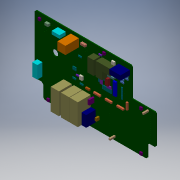
# Autodesk Inventor part: E99245-1178
Saved by Autodesk Inventor 2018 (Build 220105000, 105)
## iProperties
Created: 2004-11-23
Part Number: E99245-1178
Document SubType Name: Modeling
Designer: Autodesk, Inc.
Manufacturer: Standard
Standards Organization: Custom
Description: CONTROLER CARD, 29 SERIES
Engineer: N. GINEER
Mass: 79.5696 g
Surface Area: 565.686 cm^2
Volume: 79.5696 cm^3
Density: 1 g/cm^3
Material: Generic
Appearance: Board Outline
CAGE: 1LJX3
Dept. ID: Product Design
Description #2: ---
Finish #1: ---
Finish #2: ---
Material ID: ---
Project Number: ---
Author: Autodesk, Inc.
Autodesk Inventor part; units mm, degrees
ref_plane "YZ Plane" through (0, 0, 0) normal (1, 0, 0) x (0, 1, 0)
ref_plane "XZ Plane" through (0, 0, 0) normal (0, 1, 0) x (-1, 0, 0)
ref_plane "XY Plane" through (0, 0, 0) normal (0, 0, 1) x (1, 0, 0)
sketch "Sketch1" plane through (0, 0, 0) normal (0, 0, 1) x (1, 0, 0)
  line L0 (181.9999, 1.9998) -> (181.9999, 20)
  line L1 (181.9999, 20) -> (185.0001, 23.0001)
  line L2 (185.0001, 23.0001) -> (194.0001, 23.0001)
  line L3 (194.0001, 23.0001) -> (195.9999, 25)
  line L4 (195.9999, 25) -> (195.9999, 69.9999)
  line L5 (195.9999, 69.9999) -> (194.0001, 72.0001)
  line L6 (194.0001, 72.0001) -> (158.4998, 72.0001)
  arc A0 (156.9999, 73.5) -> (158.4998, 72.0001) centre (158.4998, 73.5) ccw
  line L7 (156.9999, 73.5) -> (156.9999, 116.0001)
  line L8 (156.9999, 116.0001) -> (155.0001, 117.9999)
  line L9 (155.0001, 117.9999) -> (1.9998, 117.9999)
  line L10 (1.9998, 117.9999) -> (0, 116.0001)
  line L11 (0, 116.0001) -> (0, 25)
  line L12 (0, 25) -> (1.9998, 23.0001)
  line L13 (1.9998, 23.0001) -> (10.9999, 23.0001)
  line L14 (10.9999, 23.0001) -> (14.0001, 20)
  line L15 (14.0001, 20) -> (14.0001, 1.9998)
  line L16 (14.0001, 1.9998) -> (15.9999, 0)
  line L17 (15.9999, 0) -> (180.0001, 0)
  line L18 (180.0001, 0) -> (181.9999, 1.9998)
  circle A1 centre (22.987, 3.9878) radius 1.7526
  circle A2 centre (172.9994, 3.9878) radius 1.7526
  circle A3 centre (172.9994, 66.9798) radius 1.7526
  circle A4 centre (113.0046, 113.9952) radius 1.7526
  circle A5 centre (8.9916, 110.0074) radius 1.7526
  circle A6 centre (137.3124, 106.68) radius 0.508
  circle A7 centre (152.2476, 106.68) radius 0.508
  circle A8 centre (103.505, 19.685) radius 0.3937
  circle A9 centre (103.505, 17.145) radius 0.3937
  circle A10 centre (94.615, 25.8826) radius 0.508
  circle A11 centre (94.615, 10.9474) radius 0.508
  circle A12 centre (83.82, 41.275) radius 0.4826
  circle A13 centre (83.82, 12.065) radius 0.4826
  circle A14 centre (95.25, 42.545) radius 0.3937
  circle A15 centre (95.25, 37.465) radius 0.3937
  circle A16 centre (69.85, 41.275) radius 0.4826
  circle A17 centre (69.85, 12.065) radius 0.4826
  circle A18 centre (61.595, 17.145) radius 0.3937
  circle A19 centre (61.595, 12.065) radius 0.3937
  circle A20 centre (53.34, 41.275) radius 0.4826
  circle A21 centre (53.34, 12.065) radius 0.4826
  circle A22 centre (100.33, 109.22) radius 0.635
  circle A23 centre (100.33, 78.74) radius 0.635
  circle A24 centre (106.045, 100.965) radius 0.635
  circle A25 centre (136.525, 100.965) radius 0.635
  circle A26 centre (113.665, 109.855) radius 0.635
  circle A27 centre (113.665, 79.375) radius 0.635
  circle A28 centre (62.23, 107.315) radius 0.4318
  circle A29 centre (67.31, 107.315) radius 0.4318
  circle A30 centre (120.65, 107.95) radius 0.3556
  circle A31 centre (120.65, 97.79) radius 0.3556
  circle A32 centre (73.66, 110.49) radius 0.5334
  circle A33 centre (87.63, 110.49) radius 0.5334
  circle A34 centre (16.51, 109.855) radius 0.508
  circle A35 centre (27.94, 109.855) radius 0.508
  circle A36 centre (55.245, 109.855) radius 0.7112
  circle A37 centre (50.165, 109.855) radius 0.7112
  circle A38 centre (37.465, 109.855) radius 0.7112
  circle A39 centre (32.385, 109.855) radius 0.7112
  circle A40 centre (127, 81.28) radius 0.4318
  circle A41 centre (127, 78.74) radius 0.4318
  circle A42 centre (127, 76.2) radius 0.4318
  circle A43 centre (127, 73.66) radius 0.4318
  circle A44 centre (127, 71.12) radius 0.4318
  circle A45 centre (127, 68.58) radius 0.4318
  circle A46 centre (127, 66.04) radius 0.4318
  circle A47 centre (134.62, 66.04) radius 0.4318
  circle A48 centre (134.62, 68.58) radius 0.4318
  circle A49 centre (134.62, 71.12) radius 0.4318
  circle A50 centre (134.62, 73.66) radius 0.4318
  circle A51 centre (134.62, 76.2) radius 0.4318
  circle A52 centre (134.62, 78.74) radius 0.4318
  circle A53 centre (134.62, 81.28) radius 0.4318
  circle A54 centre (115.57, 81.915) radius 0.4318
  circle A55 centre (115.57, 79.375) radius 0.4318
  circle A56 centre (115.57, 76.835) radius 0.4318
  circle A57 centre (115.57, 74.295) radius 0.4318
  circle A58 centre (123.19, 74.295) radius 0.4318
  circle A59 centre (123.19, 76.835) radius 0.4318
  circle A60 centre (123.19, 79.375) radius 0.4318
  circle A61 centre (123.19, 81.915) radius 0.4318
  circle A62 centre (129.413, 5.715) radius 0.4699
  circle A63 centre (183.515, 68.58) radius 0.4699
  circle A64 centre (126.365, 92.71) radius 0.4699
  circle A65 centre (131.445, 92.71) radius 0.4699
  circle A66 centre (133.985, 92.71) radius 0.4699
  circle A67 centre (186.69, 62.865) radius 0.4699
  circle A68 centre (186.69, 60.325) radius 0.4699
  circle A69 centre (186.69, 57.785) radius 0.4699
  circle A70 centre (186.69, 55.245) radius 0.4699
  circle A71 centre (186.69, 52.705) radius 0.4699
  circle A72 centre (186.69, 50.165) radius 0.4699
  circle A73 centre (186.69, 47.625) radius 0.4699
  circle A74 centre (186.69, 45.085) radius 0.4699
  circle A75 centre (186.69, 42.545) radius 0.4699
  circle A76 centre (186.69, 40.005) radius 0.4699
  circle A77 centre (186.69, 37.465) radius 0.4699
  circle A78 centre (186.69, 34.925) radius 0.4699
  circle A79 centre (186.69, 32.385) radius 0.4699
  circle A80 centre (186.69, 29.845) radius 0.4699
  circle A81 centre (81.915, 51.435) radius 0.3937
  circle A82 centre (92.075, 51.435) radius 0.3937
  circle A83 centre (147.32, 51.435) radius 0.4318
  circle A84 centre (132.08, 51.435) radius 0.4318
  circle A85 centre (128.27, 51.435) radius 0.4318
  circle A86 centre (113.03, 51.435) radius 0.4318
  circle A87 centre (109.855, 51.435) radius 0.4318
  circle A88 centre (94.615, 51.435) radius 0.4318
  circle A89 centre (150.495, 51.435) radius 0.4318
  circle A90 centre (150.495, 66.675) radius 0.4318
  circle A91 centre (120.65, 5.715) radius 0.3937
  circle A92 centre (120.65, 15.875) radius 0.3937
  circle A93 centre (138.43, 66.04) radius 0.4318
  circle A94 centre (138.43, 81.28) radius 0.4318
  circle A95 centre (101.6, 66.04) radius 0.4318
  circle A96 centre (101.6, 81.28) radius 0.4318
  circle A97 centre (120.65, 19.685) radius 0.3937
  circle A98 centre (120.65, 29.845) radius 0.3937
  circle A99 centre (60.325, 66.04) radius 0.3937
  circle A100 centre (60.325, 76.2) radius 0.3937
  circle A101 centre (120.65, 33.02) radius 0.3937
  circle A102 centre (120.65, 43.18) radius 0.3937
  circle A103 centre (117.475, 43.18) radius 0.3937
  circle A104 centre (107.315, 43.18) radius 0.3937
  circle A105 centre (8.255, 27.94) radius 0.4318
  circle A106 centre (8.255, 53.34) radius 0.4318
  circle A107 centre (26.7462, 23.495) radius 0.6604
  circle A108 centre (39.243, 23.495) radius 0.6604
  circle A109 centre (39.243, 28.4734) radius 0.6604
  circle A110 centre (26.7462, 28.4734) radius 0.6604
  circle A111 centre (32.9946, 30.48) radius 0.9144
  circle A112 centre (32.9946, 21.4884) radius 0.9144
  circle A113 centre (106.68, 85.09) radius 0.6604
  circle A114 centre (137.16, 85.09) radius 0.6604
  circle A115 centre (144.78, 73.66) radius 0.6604
  circle A116 centre (137.16, 62.23) radius 0.6604
  circle A117 centre (106.68, 62.23) radius 0.6604
  circle A118 centre (99.06, 73.66) radius 0.6604
  circle A119 centre (32.9946, 73.9902) radius 4.7498
  circle A120 centre (113.665, 102.235) radius 0.3048
  circle A121 centre (167.7416, 62.8904) radius 0.3048
  circle A122 centre (151.13, 86.36) radius 0.3048
  circle A123 centre (78.105, 66.04) radius 0.3048
  circle A124 centre (92.075, 96.52) radius 0.3048
  circle A125 centre (71.755, 53.34) radius 0.3048
  circle A126 centre (69.215, 72.39) radius 0.3048
  circle A127 centre (69.215, 74.93) radius 0.3048
  circle A128 centre (139.065, 64.135) radius 0.3048
  circle A129 centre (69.85, 67.31) radius 0.3048
  circle A130 centre (115.57, 71.755) radius 0.3048
  circle A131 centre (60.96, 62.865) radius 0.3048
  circle A132 centre (71.755, 67.31) radius 0.3048
  circle A133 centre (60.96, 60.325) radius 0.3048
  circle A134 centre (71.12, 55.88) radius 0.3048
  circle A135 centre (72.39, 71.755) radius 0.3048
  circle A136 centre (14.605, 27.94) radius 0.3048
  circle A137 centre (48.26, 101.6) radius 0.3048
  circle A138 centre (36.195, 91.44) radius 0.3048
  circle A139 centre (111.125, 108.585) radius 0.3048
  circle A140 centre (55.5752, 102.5144) radius 0.3048
  circle A141 centre (77.47, 97.79) radius 0.3048
  circle A142 centre (15.875, 95.885) radius 0.6858
  circle A143 centre (15.875, 100.965) radius 0.6858
  circle A144 centre (18.415, 98.425) radius 0.6858
  circle A145 centre (81.915, 100.33) radius 0.6858
  circle A146 centre (81.915, 105.41) radius 0.6858
  circle A147 centre (84.455, 102.87) radius 0.6858
  constraints: 148 centre point, 38 end point, 2 point on circle
extrude "example2.max_Outline" add sketch "Sketch1" along normal blind 1.5748
sketch "3.5MTH, 0_1" plane through (0, 0, 1.5748) normal (0, 0, 1) x (1, 0, 0)
  line L0 (21.082, 2.0828) -> (21.082, 5.8928)
  line L1 (21.082, 5.8928) -> (24.892, 5.8928)
  line L2 (24.892, 5.8928) -> (24.892, 2.0828)
  line L3 (24.892, 2.0828) -> (21.082, 2.0828)
  constraints: 8 end point
extrude "11_2" add sketch "3.5MTH, 0_1" along normal blind 2.54
sketch "3.5MTH, 0_3" plane through (0, 0, 1.5748) normal (0, 0, 1) x (1, 0, 0)
  line L0 (171.0944, 2.0828) -> (171.0944, 5.8928)
  line L1 (171.0944, 5.8928) -> (174.9044, 5.8928)
  line L2 (174.9044, 5.8928) -> (174.9044, 2.0828)
  line L3 (174.9044, 2.0828) -> (171.0944, 2.0828)
  constraints: 8 end point
extrude "21_4" add sketch "3.5MTH, 0_3" along normal blind 2.54
sketch "3.5MTH, 0_5" plane through (0, 0, 1.5748) normal (0, 0, 1) x (1, 0, 0)
  line L0 (171.0944, 65.0748) -> (171.0944, 68.8848)
  line L1 (171.0944, 68.8848) -> (174.9044, 68.8848)
  line L2 (174.9044, 68.8848) -> (174.9044, 65.0748)
  line L3 (174.9044, 65.0748) -> (171.0944, 65.0748)
  constraints: 8 end point
extrude "31_6" add sketch "3.5MTH, 0_5" along normal blind 2.54
sketch "3.5MTH, 0_7" plane through (0, 0, 1.5748) normal (0, 0, 1) x (1, 0, 0)
  line L0 (111.0996, 112.0902) -> (111.0996, 115.9002)
  line L1 (111.0996, 115.9002) -> (114.9096, 115.9002)
  line L2 (114.9096, 115.9002) -> (114.9096, 112.0902)
  line L3 (114.9096, 112.0902) -> (111.0996, 112.0902)
  constraints: 8 end point
extrude "41_8" add sketch "3.5MTH, 0_7" along normal blind 2.54
sketch "3.5MTH, 0_9" plane through (0, 0, 1.5748) normal (0, 0, 1) x (1, 0, 0)
  line L0 (7.0866, 108.1024) -> (7.0866, 111.9124)
  line L1 (7.0866, 111.9124) -> (10.8966, 111.9124)
  line L2 (10.8966, 111.9124) -> (10.8966, 108.1024)
  line L3 (10.8966, 108.1024) -> (7.0866, 108.1024)
  constraints: 8 end point
extrude "51_10" add sketch "3.5MTH, 0_9" along normal blind 2.54
sketch "RAD_.725X.300_LS.588_.040, 470NF_11" plane through (0, 0, 1.5748) normal (0, 0, 1) x (1, 0, 0)
  line L0 (153.67, 110.49) -> (135.89, 110.49)
  line L1 (135.89, 110.49) -> (135.89, 102.87)
  line L2 (135.89, 102.87) -> (153.67, 102.87)
  line L3 (153.67, 102.87) -> (153.67, 110.49)
  constraints: 8 end point
extrude "C1_12" add sketch "RAD_.725X.300_LS.588_.040, 470NF_11" along normal blind 15.24
sketch "SM_C_1206, 10NF_13" plane through (0, 0, 1.5748) normal (0, 0, 1) x (1, 0, 0)
  line L0 (117.602, 62.865) -> (119.888, 62.865)
  line L1 (119.888, 62.865) -> (119.888, 68.453)
  line L2 (119.888, 68.453) -> (117.602, 68.453)
  line L3 (117.602, 68.453) -> (117.602, 62.865)
  constraints: 8 end point
extrude "C2_14" add sketch "SM_C_1206, 10NF_13" along normal blind 1.27
sketch "SM_C_1206, 10NF_15" plane through (0, 0, 1.5748) normal (0, 0, 1) x (1, 0, 0)
  line L0 (105.918, 75.565) -> (103.632, 75.565)
  line L1 (103.632, 75.565) -> (103.632, 69.977)
  line L2 (103.632, 69.977) -> (105.918, 69.977)
  line L3 (105.918, 69.977) -> (105.918, 75.565)
  constraints: 8 end point
extrude "C3_16" add sketch "SM_C_1206, 10NF_15" along normal blind 1.27
sketch "SM_C_1206, 10NF_17" plane through (0, 0, 1.5748) normal (0, 0, 1) x (1, 0, 0)
  line L0 (112.268, 68.58) -> (109.982, 68.58)
  line L1 (109.982, 68.58) -> (109.982, 62.992)
  line L2 (109.982, 62.992) -> (112.268, 62.992)
  line L3 (112.268, 62.992) -> (112.268, 68.58)
  constraints: 8 end point
extrude "C4_18" add sketch "SM_C_1206, 10NF_17" along normal blind 1.27
sketch "SM_C_1206, 10NF_19" plane through (0, 0, 1.5748) normal (0, 0, 1) x (1, 0, 0)
  line L0 (115.062, 62.865) -> (117.348, 62.865)
  line L1 (117.348, 62.865) -> (117.348, 68.453)
  line L2 (117.348, 68.453) -> (115.062, 68.453)
  line L3 (115.062, 68.453) -> (115.062, 62.865)
  constraints: 8 end point
extrude "C5_20" add sketch "SM_C_1206, 10NF_19" along normal blind 1.27
sketch "SM_C_1206, 10NF_21" plane through (0, 0, 1.5748) normal (0, 0, 1) x (1, 0, 0)
  line L0 (62.23, 70.993) -> (62.23, 68.707)
  line L1 (62.23, 68.707) -> (67.818, 68.707)
  line L2 (67.818, 68.707) -> (67.818, 70.993)
  line L3 (67.818, 70.993) -> (62.23, 70.993)
  constraints: 8 end point
extrude "C6_22" add sketch "SM_C_1206, 10NF_21" along normal blind 1.27
sketch "SM_C_1206, 10NF_23" plane through (0, 0, 1.5748) normal (0, 0, 1) x (1, 0, 0)
  line L0 (62.23, 68.453) -> (62.23, 66.167)
  line L1 (62.23, 66.167) -> (67.818, 66.167)
  line L2 (67.818, 66.167) -> (67.818, 68.453)
  line L3 (67.818, 68.453) -> (62.23, 68.453)
  constraints: 8 end point
extrude "C7_24" add sketch "SM_C_1206, 10NF_23" along normal blind 1.27
sketch "SM_C_1206, 10NF_25" plane through (0, 0, 1.5748) normal (0, 0, 1) x (1, 0, 0)
  line L0 (73.66, 53.213) -> (73.66, 50.927)
  line L1 (73.66, 50.927) -> (79.248, 50.927)
  line L2 (79.248, 50.927) -> (79.248, 53.213)
  line L3 (79.248, 53.213) -> (73.66, 53.213)
  constraints: 8 end point
extrude "C8_26" add sketch "SM_C_1206, 10NF_25" along normal blind 1.27
sketch "SM_C_1206, 10NF_27" plane through (0, 0, 1.5748) normal (0, 0, 1) x (1, 0, 0)
  line L0 (136.017, 95.885) -> (138.303, 95.885)
  line L1 (138.303, 95.885) -> (138.303, 101.473)
  line L2 (138.303, 101.473) -> (136.017, 101.473)
  line L3 (136.017, 101.473) -> (136.017, 95.885)
  constraints: 8 end point
extrude "C9_28" add sketch "SM_C_1206, 10NF_27" along normal blind 1.27
sketch "RAD_.150X.100_LS.100_.031, 1NF_29" plane through (0, 0, 1.5748) normal (0, 0, 1) x (1, 0, 0)
  line L0 (102.1334, 20.7264) -> (102.1334, 16.1036)
  line L1 (102.1334, 16.1036) -> (104.8766, 16.1036)
  line L2 (104.8766, 16.1036) -> (104.8766, 20.7264)
  line L3 (104.8766, 20.7264) -> (102.1334, 20.7264)
  constraints: 8 end point
extrude "C10_30" add sketch "RAD_.150X.100_LS.100_.031, 1NF_29" along normal blind 5.08
sketch "RAD_.725X.300_LS.588_.040, 470NF_31" plane through (0, 0, 1.5748) normal (0, 0, 1) x (1, 0, 0)
  line L0 (98.425, 9.525) -> (98.425, 27.305)
  line L1 (98.425, 27.305) -> (90.805, 27.305)
  line L2 (90.805, 27.305) -> (90.805, 9.525)
  line L3 (90.805, 9.525) -> (98.425, 9.525)
  constraints: 8 end point
extrude "C11_32" add sketch "RAD_.725X.300_LS.588_.040, 470NF_31" along normal blind 15.24
sketch "RAD_1.200X.250_LS1.100_.040, 2.2UF_33" plane through (0, 0, 1.5748) normal (0, 0, 1) x (1, 0, 0)
  line L0 (77.216, 44.069) -> (90.424, 44.069)
  line L1 (90.424, 44.069) -> (90.424, 9.271)
  line L2 (90.424, 9.271) -> (77.216, 9.271)
  line L3 (77.216, 9.271) -> (77.216, 44.069)
  constraints: 8 end point
extrude "C12_34" add sketch "RAD_1.200X.250_LS1.100_.040, 2.2UF_33" along normal blind 20.828
sketch "RAD_.300X.100_LS.200_.031, 100PF_35" plane through (0, 0, 1.5748) normal (0, 0, 1) x (1, 0, 0)
  line L0 (93.98, 36.195) -> (93.98, 43.815)
  line L1 (93.98, 43.815) -> (96.52, 43.815)
  line L2 (96.52, 43.815) -> (96.52, 36.195)
  line L3 (96.52, 36.195) -> (93.98, 36.195)
  constraints: 8 end point
extrude "C13_36" add sketch "RAD_.300X.100_LS.200_.031, 100PF_35" along normal blind 8.255
sketch "RAD_1.200X.250_LS1.100_.040, 2.2UF_37" plane through (0, 0, 1.5748) normal (0, 0, 1) x (1, 0, 0)
  line L0 (63.246, 44.069) -> (76.454, 44.069)
  line L1 (76.454, 44.069) -> (76.454, 9.271)
  line L2 (76.454, 9.271) -> (63.246, 9.271)
  line L3 (63.246, 9.271) -> (63.246, 44.069)
  constraints: 8 end point
extrude "C14_38" add sketch "RAD_1.200X.250_LS1.100_.040, 2.2UF_37" along normal blind 20.828
sketch "RAD_.300X.100_LS.200_.031, 100PF_39" plane through (0, 0, 1.5748) normal (0, 0, 1) x (1, 0, 0)
  line L0 (60.325, 10.795) -> (60.325, 18.415)
  line L1 (60.325, 18.415) -> (62.865, 18.415)
  line L2 (62.865, 18.415) -> (62.865, 10.795)
  line L3 (62.865, 10.795) -> (60.325, 10.795)
  constraints: 8 end point
extrude "C15_40" add sketch "RAD_.300X.100_LS.200_.031, 100PF_39" along normal blind 8.255
sketch "RAD_1.200X.250_LS1.100_.040, 2.2UF_41" plane through (0, 0, 1.5748) normal (0, 0, 1) x (1, 0, 0)
  line L0 (46.736, 44.069) -> (59.944, 44.069)
  line L1 (59.944, 44.069) -> (59.944, 9.271)
  line L2 (59.944, 9.271) -> (46.736, 9.271)
  line L3 (46.736, 9.271) -> (46.736, 44.069)
  constraints: 8 end point
extrude "C16_42" add sketch "RAD_1.200X.250_LS1.100_.040, 2.2UF_41" along normal blind 20.828
sketch "SM_C_1206, 10NF_43" plane through (0, 0, 1.5748) normal (0, 0, 1) x (1, 0, 0)
  line L0 (120.142, 62.865) -> (122.428, 62.865)
  line L1 (122.428, 62.865) -> (122.428, 68.453)
  line L2 (122.428, 68.453) -> (120.142, 68.453)
  line L3 (120.142, 68.453) -> (120.142, 62.865)
  constraints: 8 end point
extrude "C17_44" add sketch "SM_C_1206, 10NF_43" along normal blind 1.27
sketch "SM_C_1206, 10NF_45" plane through (0, 0, 1.5748) normal (0, 0, 1) x (1, 0, 0)
  line L0 (111.252, 75.565) -> (113.538, 75.565)
  line L1 (113.538, 75.565) -> (113.538, 81.153)
  line L2 (113.538, 81.153) -> (111.252, 81.153)
  line L3 (111.252, 81.153) -> (111.252, 75.565)
  constraints: 8 end point
extrude "C18_46" add sketch "SM_C_1206, 10NF_45" along normal blind 1.27
sketch "SM_C_1206, 10NF_47" plane through (0, 0, 1.5748) normal (0, 0, 1) x (1, 0, 0)
  line L0 (114.808, 68.58) -> (112.522, 68.58)
  line L1 (112.522, 68.58) -> (112.522, 62.992)
  line L2 (112.522, 62.992) -> (114.808, 62.992)
  line L3 (114.808, 62.992) -> (114.808, 68.58)
  constraints: 8 end point
extrude "C19_48" add sketch "SM_C_1206, 10NF_47" along normal blind 1.27
sketch "SM_C_1206, 10NF_49" plane through (0, 0, 1.5748) normal (0, 0, 1) x (1, 0, 0)
  line L0 (142.748, 80.645) -> (140.462, 80.645)
  line L1 (140.462, 80.645) -> (140.462, 75.057)
  line L2 (140.462, 75.057) -> (142.748, 75.057)
  line L3 (142.748, 75.057) -> (142.748, 80.645)
  constraints: 8 end point
extrude "C20_50" add sketch "SM_C_1206, 10NF_49" along normal blind 1.27
sketch "SM_C_1206, 10NF_51" plane through (0, 0, 1.5748) normal (0, 0, 1) x (1, 0, 0)
  line L0 (67.31, 53.467) -> (67.31, 55.753)
  line L1 (67.31, 55.753) -> (61.722, 55.753)
  line L2 (61.722, 55.753) -> (61.722, 53.467)
  line L3 (61.722, 53.467) -> (67.31, 53.467)
  constraints: 8 end point
extrude "C21_52" add sketch "SM_C_1206, 10NF_51" along normal blind 1.27
sketch "SM_C_1206, 10NF_53" plane through (0, 0, 1.5748) normal (0, 0, 1) x (1, 0, 0)
  line L0 (142.748, 74.93) -> (140.462, 74.93)
  line L1 (140.462, 74.93) -> (140.462, 69.342)
  line L2 (140.462, 69.342) -> (142.748, 69.342)
  line L3 (142.748, 69.342) -> (142.748, 74.93)
  constraints: 8 end point
extrude "C22_54" add sketch "SM_C_1206, 10NF_53" along normal blind 1.27
sketch "SM_C_1206, 10NF_55" plane through (0, 0, 1.5748) normal (0, 0, 1) x (1, 0, 0)
  line L0 (142.748, 69.215) -> (140.462, 69.215)
  line L1 (140.462, 69.215) -> (140.462, 63.627)
  line L2 (140.462, 63.627) -> (142.748, 63.627)
  line L3 (142.748, 63.627) -> (142.748, 69.215)
  constraints: 8 end point
extrude "C23_56" add sketch "SM_C_1206, 10NF_55" along normal blind 1.27
sketch "SM_C_1206, 10NF_57" plane through (0, 0, 1.5748) normal (0, 0, 1) x (1, 0, 0)
  line L0 (122.682, 62.865) -> (124.968, 62.865)
  line L1 (124.968, 62.865) -> (124.968, 68.453)
  line L2 (124.968, 68.453) -> (122.682, 68.453)
  line L3 (122.682, 68.453) -> (122.682, 62.865)
  constraints: 8 end point
extrude "C24_58" add sketch "SM_C_1206, 10NF_57" along normal blind 1.27
sketch "SM_C_1206, 10NF_59" plane through (0, 0, 1.5748) normal (0, 0, 1) x (1, 0, 0)
  line L0 (99.06, 83.312) -> (99.06, 85.598)
  line L1 (99.06, 85.598) -> (93.472, 85.598)
  line L2 (93.472, 85.598) -> (93.472, 83.312)
  line L3 (93.472, 83.312) -> (99.06, 83.312)
  constraints: 8 end point
extrude "C25_60" add sketch "SM_C_1206, 10NF_59" along normal blind 1.27
sketch "SM_C_1206, 10NF_61" plane through (0, 0, 1.5748) normal (0, 0, 1) x (1, 0, 0)
  line L0 (76.4794, 88.5698) -> (76.4794, 90.8558)
  line L1 (76.4794, 90.8558) -> (70.8914, 90.8558)
  line L2 (70.8914, 90.8558) -> (70.8914, 88.5698)
  line L3 (70.8914, 88.5698) -> (76.4794, 88.5698)
  constraints: 8 end point
extrude "C26_62" add sketch "SM_C_1206, 10NF_61" along normal blind 1.27
sketch "AX_1.200X.400_.050, 10UF_63" plane through (0, 0, 1.5748) normal (0, 0, 1) x (1, 0, 0)
  line L0 (95.25, 82.8675) -> (95.25, 105.0925)
  line L1 (95.25, 105.0925) -> (105.41, 105.0925)
  line L2 (105.41, 105.0925) -> (105.41, 82.8675)
  line L3 (105.41, 82.8675) -> (95.25, 82.8675)
  constraints: 8 end point
extrude "C27_64" add sketch "AX_1.200X.400_.050, 10UF_63" along normal blind 10.16
sketch "AX_1.200X.400_.050, 10UF_65" plane through (0, 0, 1.5748) normal (0, 0, 1) x (1, 0, 0)
  line L0 (132.3975, 95.885) -> (110.1725, 95.885)
  line L1 (110.1725, 95.885) -> (110.1725, 106.045)
  line L2 (110.1725, 106.045) -> (132.3975, 106.045)
  line L3 (132.3975, 106.045) -> (132.3975, 95.885)
  constraints: 8 end point
extrude "C28_66" add sketch "AX_1.200X.400_.050, 10UF_65" along normal blind 10.16
sketch "AX_1.200X.400_.050, 10UF_67" plane through (0, 0, 1.5748) normal (0, 0, 1) x (1, 0, 0)
  line L0 (108.585, 83.5025) -> (108.585, 105.7275)
  line L1 (108.585, 105.7275) -> (118.745, 105.7275)
  line L2 (118.745, 105.7275) -> (118.745, 83.5025)
  line L3 (118.745, 83.5025) -> (108.585, 83.5025)
  constraints: 8 end point
extrude "C30_68" add sketch "AX_1.200X.400_.050, 10UF_67" along normal blind 10.16
sketch "CAPTEST, 1MF_69" plane through (0, 0, 1.5748) normal (0, 0, 1) x (1, 0, 0)
  line L0 (58.3184, 100.8634) -> (58.3184, 113.7666)
  line L1 (58.3184, 113.7666) -> (71.2216, 113.7666)
  line L2 (71.2216, 113.7666) -> (71.2216, 100.8634)
  line L3 (71.2216, 100.8634) -> (58.3184, 100.8634)
  constraints: 8 end point
extrude "C31_70" add sketch "CAPTEST, 1MF_69" along normal blind 21.59
sketch "SM_D_MLL41_12, LL4148_71" plane through (0, 0, 1.5748) normal (0, 0, 1) x (1, 0, 0)
  line L0 (106.68, 83.3374) -> (106.68, 76.3778)
  line L1 (106.68, 76.3778) -> (108.3818, 76.3778)
  line L2 (108.3818, 76.3778) -> (108.585, 76.1746)
  line L3 (108.585, 76.1746) -> (108.7882, 76.3778)
  line L4 (108.7882, 76.3778) -> (110.4646, 76.3778)
  line L5 (110.4646, 76.3778) -> (110.4646, 83.3374)
  line L6 (110.4646, 83.3374) -> (106.68, 83.3374)
  constraints: 14 end point
extrude "D1_72" add sketch "SM_D_MLL41_12, LL4148_71" along normal blind 1.651
sketch "SM_D_MLL41_12, LL4148_75" plane through (0, 0, 1.5748) normal (0, 0, 1) x (1, 0, 0)
  line L0 (135.255, 97.0026) -> (135.255, 103.9622)
  line L1 (135.255, 103.9622) -> (133.5532, 103.9622)
  line L2 (133.5532, 103.9622) -> (133.35, 104.1654)
  line L3 (133.35, 104.1654) -> (133.1468, 103.9622)
  line L4 (133.1468, 103.9622) -> (131.4704, 103.9622)
  line L5 (131.4704, 103.9622) -> (131.4704, 97.0026)
  line L6 (131.4704, 97.0026) -> (135.255, 97.0026)
  constraints: 14 end point
extrude "D3_76" add sketch "SM_D_MLL41_12, LL4148_75" along normal blind 1.651
sketch "SM_D_MLL41_12, LL4148_77" plane through (0, 0, 1.5748) normal (0, 0, 1) x (1, 0, 0)
  line L0 (139.065, 101.7524) -> (139.065, 94.7928)
  line L1 (139.065, 94.7928) -> (140.7668, 94.7928)
  line L2 (140.7668, 94.7928) -> (140.97, 94.5896)
  line L3 (140.97, 94.5896) -> (141.1732, 94.7928)
  line L4 (141.1732, 94.7928) -> (142.8496, 94.7928)
  line L5 (142.8496, 94.7928) -> (142.8496, 101.7524)
  line L6 (142.8496, 101.7524) -> (139.065, 101.7524)
  constraints: 14 end point
extrude "D4_78" add sketch "SM_D_MLL41_12, LL4148_77" along normal blind 1.651
sketch "SM_D_MLL41_12, LL4148_79" plane through (0, 0, 1.5748) normal (0, 0, 1) x (1, 0, 0)
  line L0 (119.8626, 86.995) -> (126.8222, 86.995)
  line L1 (126.8222, 86.995) -> (126.8222, 88.6968)
  line L2 (126.8222, 88.6968) -> (127.0254, 88.9)
  line L3 (127.0254, 88.9) -> (126.8222, 89.1032)
  line L4 (126.8222, 89.1032) -> (126.8222, 90.7796)
  line L5 (126.8222, 90.7796) -> (119.8626, 90.7796)
  line L6 (119.8626, 90.7796) -> (119.8626, 86.995)
  constraints: 14 end point
extrude "D5_80" add sketch "SM_D_MLL41_12, LL4148_79" along normal blind 1.651
sketch "SM_D_MLL41_12, LL4148_81" plane through (0, 0, 1.5748) normal (0, 0, 1) x (1, 0, 0)
  line L0 (94.4626, 90.17) -> (101.4222, 90.17)
  line L1 (101.4222, 90.17) -> (101.4222, 91.8718)
  line L2 (101.4222, 91.8718) -> (101.6254, 92.075)
  line L3 (101.6254, 92.075) -> (101.4222, 92.2782)
  line L4 (101.4222, 92.2782) -> (101.4222, 93.9546)
  line L5 (101.4222, 93.9546) -> (94.4626, 93.9546)
  line L6 (94.4626, 93.9546) -> (94.4626, 90.17)
  constraints: 14 end point
extrude "D8_82" add sketch "SM_D_MLL41_12, LL4148_81" along normal blind 1.651
sketch "DAX1_1N_4001-4007, 1N4002_83" plane through (0, 0, 1.5748) normal (0, 0, 1) x (1, 0, 0)
  line L0 (84.455, 108.9025) -> (84.455, 112.0775)
  line L1 (84.455, 112.0775) -> (76.835, 112.0775)
  line L2 (76.835, 112.0775) -> (76.835, 108.9025)
  line L3 (76.835, 108.9025) -> (84.455, 108.9025)
  constraints: 8 end point
extrude "D9_84" add sketch "DAX1_1N_4001-4007, 1N4002_83" along normal blind 3.556
sketch "DAX1_.450X.150_.040, SB130_85" plane through (0, 0, 1.5748) normal (0, 0, 1) x (1, 0, 0)
  line L0 (25.0825, 107.95) -> (25.0825, 111.76)
  line L1 (25.0825, 111.76) -> (19.3675, 111.76)
  line L2 (19.3675, 111.76) -> (19.3675, 107.95)
  line L3 (19.3675, 107.95) -> (25.0825, 107.95)
  constraints: 8 end point
extrude "D10_86" add sketch "DAX1_.450X.150_.040, SB130_85" along normal blind 3.81
sketch "SM_D_MLL41_12, LL4148_87" plane through (0, 0, 1.5748) normal (0, 0, 1) x (1, 0, 0)
  line L0 (117.3226, 68.58) -> (124.2822, 68.58)
  line L1 (124.2822, 68.58) -> (124.2822, 70.2818)
  line L2 (124.2822, 70.2818) -> (124.4854, 70.485)
  line L3 (124.4854, 70.485) -> (124.2822, 70.6882)
  line L4 (124.2822, 70.6882) -> (124.2822, 72.3646)
  line L5 (124.2822, 72.3646) -> (117.3226, 72.3646)
  line L6 (117.3226, 72.3646) -> (117.3226, 68.58)
  constraints: 14 end point
extrude "D11_88" add sketch "SM_D_MLL41_12, LL4148_87" along normal blind 1.651
sketch "SM_D_MLL41_12, LL4148_89" plane through (0, 0, 1.5748) normal (0, 0, 1) x (1, 0, 0)
  line L0 (106.68, 75.7174) -> (106.68, 68.7578)
  line L1 (106.68, 68.7578) -> (108.3818, 68.7578)
  line L2 (108.3818, 68.7578) -> (108.585, 68.5546)
  line L3 (108.585, 68.5546) -> (108.7882, 68.7578)
  line L4 (108.7882, 68.7578) -> (110.4646, 68.7578)
  line L5 (110.4646, 68.7578) -> (110.4646, 75.7174)
  line L6 (110.4646, 75.7174) -> (106.68, 75.7174)
  constraints: 14 end point
extrude "D12_90" add sketch "SM_D_MLL41_12, LL4148_89" along normal blind 1.651
sketch "FUSE_20X5, 1A_91" plane through (0, 0, 1.5748) normal (0, 0, 1) x (1, 0, 0)
  line L0 (50.165, 112.395) -> (37.465, 112.395)
  line L1 (37.465, 112.395) -> (37.465, 107.315)
  line L2 (37.465, 107.315) -> (50.165, 107.315)
  line L3 (50.165, 107.315) -> (50.165, 112.395)
  constraints: 8 end point
extrude "F1_92" add sketch "FUSE_20X5, 1A_91" along normal blind 10.16
sketch "DIP.100_14_W.300_L.800, CA3046_93" plane through (0, 0, 1.5748) normal (0, 0, 1) x (1, 0, 0)
  line L0 (133.35, 83.82) -> (133.35, 63.5)
  line L1 (133.35, 63.5) -> (128.27, 63.5)
  line L2 (128.27, 63.5) -> (128.27, 83.82)
  line L3 (128.27, 83.82) -> (129.54, 83.82)
  line L4 (129.54, 83.82) -> (132.08, 83.82)
  line L5 (132.08, 83.82) -> (133.35, 83.82)
  constraints: 12 end point
extrude "IC1_94" add sketch "DIP.100_14_W.300_L.800, CA3046_93" along normal blind 2.54
sketch "SOG.050_8_WG.244_L.200, CA3140_95" plane through (0, 0, 1.5748) normal (0, 0, 1) x (1, 0, 0)
  line L0 (67.945, 62.4967) -> (67.945, 60.5917)
  line L1 (67.945, 60.5917) -> (73.025, 60.5917)
  line L2 (73.025, 60.5917) -> (73.025, 62.4967)
  line L3 (73.025, 62.4967) -> (67.945, 62.4967)
  constraints: 8 end point
extrude "IC2_96" add sketch "SOG.050_8_WG.244_L.200, CA3140_95" along normal blind 1.651
sketch "DIP.100_8_W.300_L.400, LF411_97" plane through (0, 0, 1.5748) normal (0, 0, 1) x (1, 0, 0)
  line L0 (121.92, 83.185) -> (116.84, 83.185)
  line L1 (116.84, 83.185) -> (116.84, 73.025)
  line L2 (116.84, 73.025) -> (121.92, 73.025)
  line L3 (121.92, 73.025) -> (121.92, 83.185)
  constraints: 8 end point
extrude "IC3_98" add sketch "DIP.100_8_W.300_L.400, LF411_97" along normal blind 3.81
sketch "SOG.050_8_WG.244_L.200, CA3140_99" plane through (0, 0, 1.5748) normal (0, 0, 1) x (1, 0, 0)
  line L0 (104.14, 109.4867) -> (104.14, 107.5817)
  line L1 (104.14, 107.5817) -> (109.22, 107.5817)
  line L2 (109.22, 107.5817) -> (109.22, 109.4867)
  line L3 (109.22, 109.4867) -> (104.14, 109.4867)
  constraints: 8 end point
extrude "IC4_100" add sketch "SOG.050_8_WG.244_L.200, CA3140_99" along normal blind 1.651
sketch "BLKCON.100_VH_TM1SQ_W.100_1, PL,1WAY,110,V_101" plane through (0, 0, 1.5748) normal (0, 0, 1) x (1, 0, 0)
  line L0 (130.683, 6.985) -> (128.143, 6.985)
  line L1 (128.143, 6.985) -> (128.143, 4.445)
  line L2 (128.143, 4.445) -> (130.683, 4.445)
  line L3 (130.683, 4.445) -> (130.683, 6.985)
  constraints: 8 end point
extrude "PL1_102" add sketch "BLKCON.100_VH_TM1SQ_W.100_1, PL,1WAY,110,V_101" along normal blind 8.89
sketch "BLKCON.100_VH_TM1SQ_W.100_1, PL,1WAY,110,V_103" plane through (0, 0, 1.5748) normal (0, 0, 1) x (1, 0, 0)
  line L0 (184.785, 69.85) -> (182.245, 69.85)
  line L1 (182.245, 69.85) -> (182.245, 67.31)
  line L2 (182.245, 67.31) -> (184.785, 67.31)
  line L3 (184.785, 67.31) -> (184.785, 69.85)
  constraints: 8 end point
extrude "PL2_104" add sketch "BLKCON.100_VH_TM1SQ_W.100_1, PL,1WAY,110,V_103" along normal blind 8.89
sketch "BLKCON.100_VH_TM1SQ_W.100_4.3, HEADER 4_3_105" plane through (0, 0, 1.5748) normal (0, 0, 1) x (1, 0, 0)
  line L0 (135.255, 93.98) -> (125.095, 93.98)
  line L1 (125.095, 93.98) -> (125.095, 91.44)
  line L2 (125.095, 91.44) -> (135.255, 91.44)
  line L3 (135.255, 91.44) -> (135.255, 93.98)
  constraints: 8 end point
extrude "PL3_106" add sketch "BLKCON.100_VH_TM1SQ_W.100_4.3, HEADER 4_3_105" along normal blind 8.255
sketch "BLKCON.100_VH_TM1SQ_W.100_14, HEADER 14_107" plane through (0, 0, 0) normal (0, 0, 1) x (1, 0, 0)
  line L0 (185.42, 28.575) -> (185.42, 64.135)
  line L1 (185.42, 64.135) -> (187.96, 64.135)
  line L2 (187.96, 64.135) -> (187.96, 28.575)
  line L3 (187.96, 28.575) -> (185.42, 28.575)
  constraints: 8 end point
extrude "PL4_108" add sketch "BLKCON.100_VH_TM1SQ_W.100_14, HEADER 14_107" against normal blind 2.54
sketch "AX_.400X.100_.031, 330K_109" plane through (0, 0, 1.5748) normal (0, 0, 1) x (1, 0, 0)
  line L0 (83.82, 50.165) -> (83.82, 51.435)
  line L1 (83.82, 51.435) -> (83.82, 52.705)
  line L2 (83.82, 52.705) -> (90.17, 52.705)
  line L3 (90.17, 52.705) -> (90.17, 51.435)
  line L4 (90.17, 51.435) -> (90.17, 50.165)
  line L5 (90.17, 50.165) -> (83.82, 50.165)
  constraints: 12 end point
extrude "R1_110" add sketch "AX_.400X.100_.031, 330K_109" along normal blind 2.54
sketch "AX_.600X.100_.034, 33M_111" plane through (0, 0, 1.5748) normal (0, 0, 1) x (1, 0, 0)
  line L0 (134.3025, 52.705) -> (134.3025, 50.165)
  line L1 (134.3025, 50.165) -> (145.0975, 50.165)
  line L2 (145.0975, 50.165) -> (145.0975, 52.705)
  line L3 (145.0975, 52.705) -> (134.3025, 52.705)
  constraints: 8 end point
extrude "R2_112" add sketch "AX_.600X.100_.034, 33M_111" along normal blind 2.54
sketch "AX_.600X.100_.034, 33M_113" plane through (0, 0, 1.5748) normal (0, 0, 1) x (1, 0, 0)
  line L0 (115.2525, 52.705) -> (115.2525, 50.165)
  line L1 (115.2525, 50.165) -> (126.0475, 50.165)
  line L2 (126.0475, 50.165) -> (126.0475, 52.705)
  line L3 (126.0475, 52.705) -> (115.2525, 52.705)
  constraints: 8 end point
extrude "R3_114" add sketch "AX_.600X.100_.034, 33M_113" along normal blind 2.54
sketch "AX_.600X.100_.034, 33M_115" plane through (0, 0, 1.5748) normal (0, 0, 1) x (1, 0, 0)
  line L0 (96.8375, 52.705) -> (96.8375, 50.165)
  line L1 (96.8375, 50.165) -> (107.6325, 50.165)
  line L2 (107.6325, 50.165) -> (107.6325, 52.705)
  line L3 (107.6325, 52.705) -> (96.8375, 52.705)
  constraints: 8 end point
extrude "R4_116" add sketch "AX_.600X.100_.034, 33M_115" along normal blind 2.54
sketch "SM_R_1206, 30K_119" plane through (0, 0, 1.5748) normal (0, 0, 1) x (1, 0, 0)
  line L0 (144.78, 86.487) -> (144.78, 88.773)
  line L1 (144.78, 88.773) -> (139.192, 88.773)
  line L2 (139.192, 88.773) -> (139.192, 86.487)
  line L3 (139.192, 86.487) -> (144.78, 86.487)
  constraints: 8 end point
extrude "R6_120" add sketch "SM_R_1206, 30K_119" along normal blind 1.27
sketch "SM_R_1206, 30K_121" plane through (0, 0, 1.5748) normal (0, 0, 1) x (1, 0, 0)
  line L0 (151.765, 94.742) -> (151.765, 97.028)
  line L1 (151.765, 97.028) -> (146.177, 97.028)
  line L2 (146.177, 97.028) -> (146.177, 94.742)
  line L3 (146.177, 94.742) -> (151.765, 94.742)
  constraints: 8 end point
extrude "R7_122" add sketch "SM_R_1206, 30K_121" along normal blind 1.27
sketch "AX_.600X.100_.034, 33M_123" plane through (0, 0, 1.5748) normal (0, 0, 1) x (1, 0, 0)
  line L0 (151.765, 64.4525) -> (149.225, 64.4525)
  line L1 (149.225, 64.4525) -> (149.225, 53.6575)
  line L2 (149.225, 53.6575) -> (151.765, 53.6575)
  line L3 (151.765, 53.6575) -> (151.765, 64.4525)
  constraints: 8 end point
extrude "R8_124" add sketch "AX_.600X.100_.034, 33M_123" along normal blind 2.54
sketch "SM_R_1206, 30K_127" plane through (0, 0, 1.5748) normal (0, 0, 1) x (1, 0, 0)
  line L0 (144.78, 90.297) -> (144.78, 92.583)
  line L1 (144.78, 92.583) -> (139.192, 92.583)
  line L2 (139.192, 92.583) -> (139.192, 90.297)
  line L3 (139.192, 90.297) -> (144.78, 90.297)
  constraints: 8 end point
extrude "R10_128" add sketch "SM_R_1206, 30K_127" along normal blind 1.27
sketch "SM_R_1206, 30K_129" plane through (0, 0, 1.5748) normal (0, 0, 1) x (1, 0, 0)
  line L0 (151.765, 98.552) -> (151.765, 100.838)
  line L1 (151.765, 100.838) -> (146.177, 100.838)
  line L2 (146.177, 100.838) -> (146.177, 98.552)
  line L3 (146.177, 98.552) -> (151.765, 98.552)
  constraints: 8 end point
extrude "R11_130" add sketch "SM_R_1206, 30K_129" along normal blind 1.27
sketch "VRES36, 500R_135" plane through (0, 0, 1.5748) normal (0, 0, 1) x (1, 0, 0)
  line L0 (78.8416, 64.643) -> (73.914, 64.643)
  line L1 (73.914, 64.643) -> (73.914, 58.8137)
  line L2 (73.914, 58.8137) -> (78.8416, 58.8137)
  line L3 (78.8416, 58.8137) -> (78.8416, 64.643)
  constraints: 8 end point
extrude "R14_136" add sketch "VRES36, 500R_135" along normal blind 2.54
sketch "VRES36, 500R_137" plane through (0, 0, 1.5748) normal (0, 0, 1) x (1, 0, 0)
  line L0 (125.6284, 104.902) -> (130.556, 104.902)
  line L1 (130.556, 104.902) -> (130.556, 110.7313)
  line L2 (130.556, 110.7313) -> (125.6284, 110.7313)
  line L3 (125.6284, 110.7313) -> (125.6284, 104.902)
  constraints: 8 end point
extrude "R15_138" add sketch "VRES36, 500R_137" along normal blind 2.54
sketch "AX_1.000X.325_.037, 30R_205" plane through (0, 0, 1.5748) normal (0, 0, 1) x (1, 0, 0)
  line L0 (12.3825, 50.8) -> (12.3825, 30.48)
  line L1 (12.3825, 30.48) -> (4.1275, 30.48)
  line L2 (4.1275, 30.48) -> (4.1275, 50.8)
  line L3 (4.1275, 50.8) -> (12.3825, 50.8)
  constraints: 8 end point
extrude "R49_206" add sketch "AX_1.000X.325_.037, 30R_205" along normal blind 8.255
body "Solid1"
